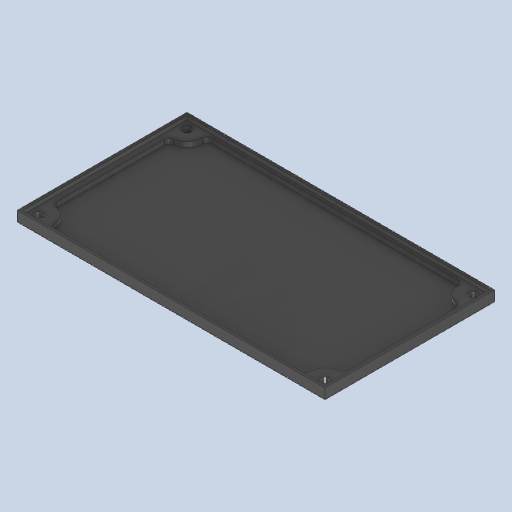
# Autodesk Inventor part: MainBoard_cover
Saved by Autodesk Inventor 2022.3 (Build 263350000, 350)
## iProperties
Part Number: MainBoard_cover
Material: 一般
Document SubType Name: Modeling
Designer: Masato Kubotera
Density: 1 g/cm^3
Appearance: 濃い灰色
Description: PLA
Mass: 6.13737 g
Surface Area: 193.634 cm^2
Volume: 6.13737 cm^3
Author: Masato Kubotera
Autodesk Inventor part; units mm, degrees
ref_plane "YZ Plane" through (0, 0, 0) normal (1, 0, 0) x (0, 1, 0)
ref_plane "XZ Plane" through (0, 0, 0) normal (0, 1, 0) x (-1, 0, 0)
ref_plane "XY Plane" through (0, 0, 0) normal (0, 0, 1) x (1, 0, 0)
derived "MainBoard.ipt"
sketch "スケッチ3" plane through (0, 0, -88.5) normal (0, 0, 1) x (1, 0, 0)
  line L0 (20.25, -135) -> (20.25, 0)
  line L1 (-83.25, 0) -> (-83.25, -135)
  line L2 (-31.5, -135) -> (-31.5, 0) construction
  line L3 (-83.25, -67.5) -> (20.25, -67.5) construction
  line L4 (-52.45, 1.4849) -> (-52.45, 5)
  line L5 (-52.45, 5) -> (-10.55, 5)
  line L6 (-10.55, 5) -> (-10.55, 1.4849)
  arc A0 (-53.9349, 0) -> (-52.45, 1.4849) centre (-53.1925, 0.7425) ccw
  arc A1 (-10.55, 1.4849) -> (-9.0651, 0) centre (-9.8075, 0.7425) ccw
  line L7 (-53.9349, 0) -> (-83.25, 0)
  line L8 (20.25, 0) -> (-9.0651, 0)
  line L9 (-10.55, 0) -> (-52.45, 0)
  line L10 (-52.45, -136.4849) -> (-52.45, -140)
  line L11 (-52.45, -140) -> (-10.55, -140)
  line L12 (-10.55, -140) -> (-10.55, -136.4849)
  arc A2 (-52.45, -136.4849) -> (-53.9349, -135) centre (-53.1925, -135.7425) ccw
  arc A3 (-9.0651, -135) -> (-10.55, -136.4849) centre (-9.8075, -135.7425) ccw
  line L13 (-53.9349, -135) -> (-83.25, -135)
  line L14 (20.25, -135) -> (-9.0651, -135)
  line L15 (-10.55, -135) -> (-52.45, -135)
  line L16 (15.5, -127.5) -> (-49.5, -127.5) construction
  line L17 (-49.5, -127.5) -> (-49.5, -7.5) construction
  line L18 (-49.5, -7.5) -> (15.5, -7.5) construction
  line L19 (15.5, -7.5) -> (15.5, -127.5) construction
  line L20 (15.5, -127.5) -> (-49.5, -7.5) construction
  line L21 (-49.5, -127.5) -> (15.5, -7.5) construction
  line L22 (-48.5, -116.5) -> (-48.5, -18.5)
  line L23 (-38.5627, -9.5) -> (4.5627, -9.5)
  line L24 (12.5, -10.5) -> (-46.5, -10.5) construction
  line L25 (-46.5, -10.5) -> (-46.5, -124.5) construction
  line L26 (-46.5, -124.5) -> (12.5, -124.5) construction
  line L27 (12.5, -124.5) -> (12.5, -10.5) construction
  line L28 (12.5, -10.5) -> (-46.5, -124.5) construction
  line L29 (-46.5, -10.5) -> (12.5, -124.5) construction
  circle A4 centre (12.5, -10.5) radius 2
  circle A5 centre (-46.5, -10.5) radius 2
  arc A6 (-46.5, -16.5) -> (-40.5471, -11.25) centre (-46.5, -10.5) ccw
  arc A7 (6.5471, -11.25) -> (12.5, -16.5) centre (12.5, -10.5) ccw
  line L30 (14.5, -18.5) -> (14.5, -116.5)
  line L31 (-17, -7.5) -> (-17, -127.5) construction
  line L32 (-76.25, -65) -> (-56.5, -65)
  line L33 (-54.5, -63) -> (-54.5, -7)
  line L34 (-56.5, -5) -> (-76.25, -5)
  line L35 (-78.25, -7) -> (-78.25, -63)
  arc A8 (-78.25, -63) -> (-76.25, -65) centre (-76.25, -63) ccw
  arc A9 (-56.5, -65) -> (-54.5, -63) centre (-56.5, -63) ccw
  arc A10 (-54.5, -7) -> (-56.5, -5) centre (-56.5, -7) ccw
  arc A11 (-76.25, -5) -> (-78.25, -7) centre (-76.25, -7) ccw
  arc A12 (-46.5, -16.5) -> (-48.5, -18.5) centre (-46.5, -18.5) ccw
  arc A13 (-38.5627, -9.5) -> (-40.5471, -11.25) centre (-38.5627, -11.5) ccw
  arc A14 (6.5471, -11.25) -> (4.5627, -9.5) centre (4.5627, -11.5) ccw
  arc A15 (14.5, -18.5) -> (12.5, -16.5) centre (12.5, -18.5) ccw
  line L36 (-38.5627, -125.5) -> (4.5627, -125.5)
  circle A16 centre (12.5, -124.5) radius 2
  circle A17 centre (-46.5, -124.5) radius 2
  arc A18 (-40.5471, -123.75) -> (-46.5, -118.5) centre (-46.5, -124.5) ccw
  arc A19 (12.5, -118.5) -> (6.5471, -123.75) centre (12.5, -124.5) ccw
  line L37 (-76.25, -70) -> (-56.5, -70)
  line L38 (-54.5, -72) -> (-54.5, -128)
  line L39 (-56.5, -130) -> (-76.25, -130)
  line L40 (-78.25, -128) -> (-78.25, -72)
  arc A20 (-76.25, -70) -> (-78.25, -72) centre (-76.25, -72) ccw
  arc A21 (-54.5, -72) -> (-56.5, -70) centre (-56.5, -72) ccw
  arc A22 (-56.5, -130) -> (-54.5, -128) centre (-56.5, -128) ccw
  arc A23 (-78.25, -128) -> (-76.25, -130) centre (-76.25, -128) ccw
  arc A24 (-48.5, -116.5) -> (-46.5, -118.5) centre (-46.5, -116.5) ccw
  arc A25 (-40.5471, -123.75) -> (-38.5627, -125.5) centre (-38.5627, -123.5) ccw
  arc A26 (4.5627, -125.5) -> (6.5471, -123.75) centre (4.5627, -123.5) ccw
  arc A27 (12.5, -118.5) -> (14.5, -116.5) centre (12.5, -116.5) ccw
  point P0 (0, 0)
  point P1 (-31.5, -67.5)
  point P2 (-17, -67.5)
  point P3 (-48.5, -16.1569)
  point P4 (-40.5839, -9.5)
  point P5 (6.5839, -9.5)
  point P6 (14.5, -16.1569)
ref_plane "作業平面1" through (20.25, 0, -88.5) normal (0, 0, -1) x (0, -1, 0)
sketch "スケッチ4" plane through (20.25, 0, -88.5) normal (0, 0, -1) x (0, -1, 0)
  line L0 (6.25, 71) -> (128.75, 71)
  line L1 (128.75, 71) -> (128.75, 3.5)
  line L2 (128.75, 3.5) -> (6.25, 3.5)
  line L3 (6.25, 3.5) -> (6.25, 71)
  line L4 (6.25, 71) -> (128.75, 3.5) construction
  line L5 (128.75, 71) -> (6.25, 3.5) construction
  line L6 (7.25, 70) -> (127.75, 70)
  line L7 (127.75, 70) -> (127.75, 4.5)
  line L8 (127.75, 4.5) -> (7.25, 4.5)
  line L9 (7.25, 4.5) -> (7.25, 70)
  line L10 (7.25, 70) -> (127.75, 4.5) construction
  line L11 (127.75, 70) -> (7.25, 4.5) construction
  line L12 (7.5, 4.75) -> (127.5, 4.75) construction
  line L13 (7.5, 69.75) -> (7.5, 4.75) construction
  circle A0 centre (10.5, 7.75) radius 1.75
  circle A1 centre (10.5, 66.75) radius 1.75
  circle A2 centre (124.5, 7.75) radius 1.75
  circle A3 centre (124.5, 66.75) radius 1.75
  line L14 (9.5, 58.8127) -> (9.5, 15.6873) projected
  arc A4 (9.5, 15.6873) -> (11.25, 13.7029) centre (11.5, 15.6873) ccw projected
  arc A5 (16.5, 7.75) -> (11.25, 13.7029) centre (10.5, 7.75) ccw projected
  arc A6 (16.5, 7.75) -> (18.5, 5.75) centre (18.5, 7.75) ccw projected
  arc A7 (11.25, 60.7971) -> (9.5, 58.8127) centre (11.5, 58.8127) ccw projected
  arc A8 (11.25, 60.7971) -> (16.5, 66.75) centre (10.5, 66.75) ccw projected
  arc A9 (18.5, 68.75) -> (16.5, 66.75) centre (18.5, 66.75) ccw projected
  line L15 (116.5, 68.75) -> (18.5, 68.75) projected
  arc A10 (118.5, 66.75) -> (116.5, 68.75) centre (116.5, 66.75) ccw projected
  arc A11 (118.5, 66.75) -> (123.75, 60.7971) centre (124.5, 66.75) ccw projected
  arc A12 (125.5, 58.8127) -> (123.75, 60.7971) centre (123.5, 58.8127) ccw projected
  line L16 (125.5, 58.8127) -> (125.5, 15.6873) projected
  arc A13 (123.75, 13.7029) -> (125.5, 15.6873) centre (123.5, 15.6873) ccw projected
  arc A14 (123.75, 13.7029) -> (118.5, 7.75) centre (124.5, 7.75) ccw projected
  arc A15 (116.5, 5.75) -> (118.5, 7.75) centre (116.5, 7.75) ccw projected
  line L17 (18.5, 5.75) -> (116.5, 5.75) projected
  point P0 (0, 20.25)
  point P1 (67.5, 37.25)
  point P2 (67.5, 37.25)
  point P3 (67.5, 37.25)
  point P4 (67.5, 37.25)
  dimension "d5" = 1
  dimension "d6" = 1
  dimension "d7" = 0.25
  dimension "d8" = 0.25
  dimension "d11" = 3.5
  dimension "d12" = 3.5
  dimension "d13" = 3.5
  dimension "d14" = 3.5
  constraints: 24 end point, 6 midpoint, 5 coincident, 4 centre point, 4 parallel, 2 horizontal, 2 perpendicular
  measures "d5" distance between parallel lines of L2 L8
  measures "d6" distance between parallel lines of L3 L9
  measures "d7" distance between parallel lines of L8 L12
  measures "d8" distance between parallel lines of L13 L9
  measures "d11" diameter of A0
  measures "d12" diameter of A1
  measures "d13" diameter of A2
  measures "d14" diameter of A3
extrude "押し出し1" add sketch "スケッチ4" against normal blind 4 contours L0 L1 L2 L3
extrude "押し出し2" add sketch "スケッチ4" against normal blind 2.4 contours L6 L7 L8 L9
extrude "押し出し3" add sketch "スケッチ3" along normal blind 0.4 contours L22 A12 A6 A13 L23 A14 A7 A15 L30 A27 A19 A26 L36 A25 A18 A24
equation "\"d6\" = d5"
equation "\"d8\" = d7"
equation "\"d12\" = d11"
equation "\"d13\" = d11"
equation "\"d14\" = d11"
